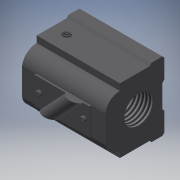
# Autodesk Inventor part: BNT 2010-2.6 Nut
Saved by Autodesk Inventor 2016 (Build 200138000, 138)
## iProperties
Category: PARTsolutions
Company: THK
Created: 2017-05-16
Part Number: BNT 2010-2.6 Nut
Catalog Web Link: www.cadenas.de
Description: BNT Nut-
Vendor: THK
Document SubType Name: Modeling
Designer: psAdmin
Manufacturer: THK
Mass: 82.4787 g
Surface Area: 175.198 cm^2
Volume: 82.4787 cm^3
Density: 1 g/cm^3
Material: Generic
Appearance: PSOLRGB-192-192-192
PSOL_IDENT_0: {$CADENAS_DATA\23d-libs\thk\fed_screw\ball_screw\ball_screw\standard_lead_rbs\bnt\bnt_nut.prj},176 {
PSOL_IDENT_1: VTYP=3D},{NB=BNT 2010-2.6 Nut},{LINA=BNT 2010-2.6 Nut},{NN=BNT Nut},{DATE=08.03.2011 04:19:39},{GEOM
PSOL_IDENT_2: DATE=23.11.2007 13:11:00},{VERSION=},{LINEID=290},{LINESUBID=-1},{WBVAR=}  {NB=BNT 2010-2.6 Nut},{LI
PSOL_IDENT_3: NA=BNT 2010-2.6 Nut},{KT=DUMMY},{MN=BNT 2010-2.6},{L=58.000},{EL=2102.000},{W=48.000},{F=18.000},{B=
PSOL_IDENT_4: 35.000},{C=35.000},{W1=24.000},{T=9.000},{M=46.000},{NDM=6.000},{KDM=4.917},{SL=10.000},{N1=10.000},
PSOL_IDENT_5: {N2=2.000},{A=6.000},{M1=41.400},{X1=1.440},{X2=20.700},{R1=10.170},{X3=4.560},{ANG=47.0},{DK=4.000}
PSOL_IDENT_6: ,{Y=1.770},{X4=0.300},{SD=20},{SL2=10.000},{Y2=14.560}
NN: BNT Nut
NB: BNT 2010-2.6 Nut
NBSYN: $MN. Nut
LINA: BNT 2010-2.6 Nut
MN: BNT 2010-2.6
L: 58.000
EL: 2102.000
W: 48.000
F: 18.000
B: 35.000
C: 35.000
W1: 24.000
T: 9.000
M: 46.000
NDM: 6.000
KDM: 4.917
SL: 10.000
N1: 10.000
N2: 2.000
A: 6.000
M1: 41.400
X1: 1.440
X2: 20.700
R1: 10.170
X3: 4.560
ANG: 47.0
DK: 4.000
Y: 1.770
X4: 0.300
SD: 20
SL2: 10.000
Y2: 14.560
SUPPLIER: THK
ARTICLENO: BNT 2010-2.6 Nut
BOMINFO: BNT 2010-2.6 Nut
CREATOR: CADENAS GmbH
Title: BNT 2010-2.6 Nut
Author: Cadenas PARTsolutions
Autodesk Inventor part; units mm, degrees
sketch "Sketch_1" plane through (0, 0, 0) normal (1, 0, 0) x (0, 1, 0)
  line L0 (16.56, 24) -> (9, 24)
  line L1 (9, 24) -> (7.56, 22.56)
  line L2 (7.56, 22.56) -> (-13.14, 22.56)
  line L3 (-13.14, 22.56) -> (-13.14, 18)
  arc A0 (-13.14, 18) -> (-23.4, 9.44) centre (-13.3579, 7.8323) ccw
  line L4 (-23.4, 9.44) -> (-23.4, -9.44)
  arc A1 (-23.4, -9.44) -> (-13.14, -18) centre (-13.3579, -7.8323) ccw
  line L5 (-13.14, -18) -> (-13.14, -22.56)
  line L6 (-13.14, -22.56) -> (7.56, -22.56)
  line L7 (7.56, -22.56) -> (9, -24)
  line L8 (9, -24) -> (16.56, -24)
  line L9 (16.56, -24) -> (18, -22.56)
  line L10 (18, -22.56) -> (18, -9.44)
  line L11 (18, -9.44) -> (16.56, -8)
  line L12 (16.56, -8) -> (16.56, 8)
  line L13 (16.56, 8) -> (18, 9.44)
  line L14 (18, 9.44) -> (18, 22.56)
  line L15 (18, 22.56) -> (16.56, 24)
  circle A2 centre (0, 0) radius 10
  constraints: 32 end point, 4 point on circle, 3 centre point
extrude "Extrusion1" add sketch "Sketch_1" along normal blind 58
sketch "Sketch_2" plane through (29, 0, 0) normal (0.682, 0, 0.7314) x (0.7314, 0, -0.682)
  line L0 (-29, -24.55) -> (-4.4539, -24.55)
  arc A0 (-4.4539, -24.55) -> (4.4539, -24.55) centre (0, -23.4) ccw
  line L1 (4.4539, -24.55) -> (29, -24.55)
  line L2 (29, -24.55) -> (29, -23.4)
  line L3 (29, -23.4) -> (-29, -23.4)
  line L4 (-29, -23.4) -> (-29, -24.55)
  constraints: 10 end point, 2 point on circle, 1 centre point
extrude "Extrusion2" add sketch "Sketch_2" along normal mid plane 58
sketch "Sketch_3" plane through (0, -23.4, 0) normal (0, 1, 0) x (1, 0, 0)
  line L0 (-29, -58) -> (87, -58)
  line L1 (87, -58) -> (87, 58)
  line L2 (87, 58) -> (-29, 58)
  line L3 (-29, 58) -> (-29, -58)
  line L4 (9.6667, -9.44) -> (48.3333, -9.44)
  line L5 (48.3333, -9.44) -> (48.3333, 9.44)
  line L6 (48.3333, 9.44) -> (9.6667, 9.44)
  line L7 (9.6667, 9.44) -> (9.6667, -9.44)
  constraints: 16 end point
extrude "Extrusion3" cut sketch "Sketch_3" against normal blind 4.6
sketch "Sketch_4" plane through (0, 0, 0) normal (0, 0, 1) x (1, 0, 0)
  line L0 (13.4367, -26.15) -> (13.4367, -24.55)
  line L1 (13.4367, -24.55) -> (15.4367, -24.55)
  line L2 (15.4367, -24.55) -> (15.4367, -25.75)
  arc A0 (15.0367, -26.15) -> (15.4367, -25.75) centre (15.0367, -25.75) ccw
  line L3 (15.0367, -26.15) -> (13.4367, -26.15)
  line L4 (13.4367, -26.15) -> (13.4367, -24.55)
  constraints: 10 end point, 2 point on circle, 1 centre point
revolve "Revolution1" add sketch "Sketch_4" angle 360 about axis through (13.4367, -26.15, 0) along (0, -1, 0)
sketch "Sketch_5" plane through (0, 0, 0) normal (0, 0, 1) x (1, 0, 0)
  line L0 (44.5633, -26.15) -> (44.5633, -24.55)
  line L1 (44.5633, -24.55) -> (46.5633, -24.55)
  line L2 (46.5633, -24.55) -> (46.5633, -25.75)
  arc A0 (46.1633, -26.15) -> (46.5633, -25.75) centre (46.1633, -25.75) ccw
  line L3 (46.1633, -26.15) -> (44.5633, -26.15)
  line L4 (44.5633, -26.15) -> (44.5633, -24.55)
  constraints: 10 end point, 2 point on circle, 1 centre point
revolve "Revolution2" add sketch "Sketch_5" angle 360 about axis through (44.5633, -26.15, 0) along (0, -1, 0)
sketch "Sketch_6" plane through (0, -26.15, 0) normal (0, 1, 0) x (1, 0, 0)
  line L0 (43.5633, 0.15) -> (43.5633, -0.15)
  line L1 (43.5633, -0.15) -> (44.4133, -0.15)
  line L2 (44.4133, -0.15) -> (44.4133, -1)
  line L3 (44.4133, -1) -> (44.7133, -1)
  line L4 (44.7133, -1) -> (44.7133, -0.15)
  line L5 (44.7133, -0.15) -> (45.5633, -0.15)
  line L6 (45.5633, -0.15) -> (45.5633, 0.15)
  line L7 (45.5633, 0.15) -> (44.7133, 0.15)
  line L8 (44.7133, 0.15) -> (44.7133, 1)
  line L9 (44.7133, 1) -> (44.4133, 1)
  line L10 (44.4133, 1) -> (44.4133, 0.15)
  line L11 (44.4133, 0.15) -> (43.5633, 0.15)
  constraints: 24 end point
extrude "Extrusion4" cut sketch "Sketch_6" along normal blind 0.8
sketch "Sketch_7" plane through (0, -26.15, 0) normal (0, 1, 0) x (1, 0, 0)
  line L0 (12.4367, 0.15) -> (12.4367, -0.15)
  line L1 (12.4367, -0.15) -> (13.2867, -0.15)
  line L2 (13.2867, -0.15) -> (13.2867, -1)
  line L3 (13.2867, -1) -> (13.5867, -1)
  line L4 (13.5867, -1) -> (13.5867, -0.15)
  line L5 (13.5867, -0.15) -> (14.4367, -0.15)
  line L6 (14.4367, -0.15) -> (14.4367, 0.15)
  line L7 (14.4367, 0.15) -> (13.5867, 0.15)
  line L8 (13.5867, 0.15) -> (13.5867, 1)
  line L9 (13.5867, 1) -> (13.2867, 1)
  line L10 (13.2867, 1) -> (13.2867, 0.15)
  line L11 (13.2867, 0.15) -> (12.4367, 0.15)
  constraints: 24 end point
extrude "Extrusion5" cut sketch "Sketch_7" along normal blind 0.8
sketch "Sketch8" plane through (0, -13.14, 22.56) normal (0, 0, 1) x (1, 0, 0)
  point P0 (10, 11.14)
hole "Hole1" at (10, -2, 22.56) direction (0, 0, -1) diameter 4.917 depth 14.1406 tip angle 120 countersink diameter 6 countersink angle 90 thread size "M6x1" class "6H" standard "ISO Metric profile"
sketch "Sketch9" plane through (0, 18, -9.44) normal (0, 1, 0) x (1, 0, 0)
  point P0 (11.5, 8.06)
hole "Hole2" at (11.5, 18, -17.5) direction (0, -1, 0) diameter 4.917 depth 13.1406 tip angle 120 countersink diameter 6 countersink angle 90 thread size "M6x1" class "6H" standard "ISO Metric profile"
pattern_linear "Rectangular Pattern1" count 2 spacing 35 along (1, 0, 0) count 2 spacing 35 along (0, 0, 1) of "Hole2"
ref_plane "bnt_nut_1_XY" through (0, 0, 0) normal (1, 0, 0) x (0, 0, -1)
ref_plane "bnt_nut_1_YZ" through (0, 0, 0) normal (0, 0, -1) x (0, 1, 0)
ref_plane "bnt_nut_1_ZX" through (0, 0, 0) normal (0, 1, 0) x (1, 0, 0)
thread "Thread1" size "M20x2.5" class "6H" standard "ANSI Metric M Profile" full length
body "Solid1"
